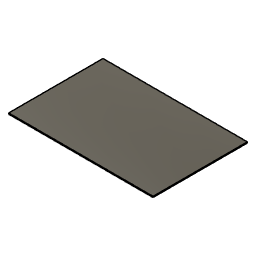
openbook_3D (Autodesk Fusion 360 archive; units mm, degrees)
design "screen"
Autodesk Fusion 360 part; units mm, degrees
box "BoxPrimitive1" add length 111.2 width 170.2 height 1.18 placed x (0, -1, 0) y (1, 0, 0) z (0, 0, 1) at (0.2, 0, 0)

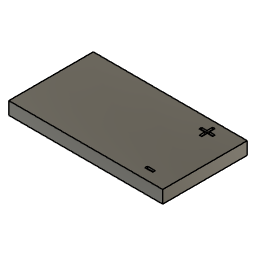
design "Battery"
part number: Configuration 1
Autodesk Fusion 360 part; units mm, degrees
box "BoxPrimitive1" add length 42 width 76.5 height 6.3 placed x (0, -1, 0) y (1, 0, 0) z (0, 0, 1) at (-66.5, 0, 0)
sketch "Sketch3" plane through (0, 0, 0) normal (0, 0, 1) x (1, 0, 0)
sketch "Sketch4" plane through (0, 0, 6.3) normal (0, 0, 1) x (-1, 0, 0)
  line L0 (66.5, 42) -> (-10, 42)
  line L1 (-10, 42) -> (-10, 0)
  line L2 (-10, 0) -> (66.5, 0)
  line L3 (66.5, 0) -> (66.5, 42)
  line L4 (0.5292, 2.4571) -> (7.6329, 2.6236) construction
  line L5 (7.6329, 2.6236) -> (7.4708, 9.5429) construction
  line L6 (7.4708, 9.5429) -> (0.3671, 9.3764) construction
  line L7 (0.3671, 9.3764) -> (0.5292, 2.4571) construction
  line L8 (1, 31) -> (8, 31) construction
  line L9 (8, 31) -> (8, 37) construction
  line L10 (8, 37) -> (1, 37) construction
  line L11 (1, 37) -> (1, 31) construction
  dimension "d8" = 10
  dimension "d9" = 10
  text T0 "+" font "Arial" height 10 align left top in box 7.1056 x 6.9211 at (0.5292, 2.4571) x (0.999726, 0.023427) y (-0.023427, 0.999726) spacing 1 kerned
extrude "Extrude1" cut sketch "Sketch4" against normal blind 1 text T0
sketch "Sketch5" plane through (0, 0, 6.3) normal (0, 0, 1) x (-1, 0, 0)
  line L0 (4.338, 5.6007) -> (4.4022, 2.8593)
  line L1 (4.4022, 2.8593) -> (3.2429, 2.8321)
  line L2 (3.2429, 2.8321) -> (3.1787, 5.5735)
  line L3 (3.1787, 5.5735) -> (0.4577, 5.5098)
  line L4 (0.4577, 5.5098) -> (0.4309, 6.6554)
  line L5 (0.4309, 6.6554) -> (3.1518, 6.7192)
  line L6 (3.1518, 6.7192) -> (3.088, 9.4401)
  line L7 (3.088, 9.4401) -> (4.2473, 9.4673)
  line L8 (4.2473, 9.4673) -> (4.3111, 6.7464)
  line L9 (4.3111, 6.7464) -> (7.0321, 6.8101)
  line L10 (7.0321, 6.8101) -> (7.0589, 5.6645)
  line L11 (7.0589, 5.6645) -> (4.338, 5.6007)
  line L12 (66.5, 42) -> (-10, 42)
  line L13 (-10, 42) -> (-10, 0)
  line L14 (-10, 0) -> (66.5, 0)
  line L15 (66.5, 0) -> (66.5, 42)
  line L16 (0, 30) -> (9, 30) construction
  line L17 (9, 30) -> (9, 37) construction
  line L18 (9, 37) -> (0, 37) construction
  line L19 (0, 37) -> (0, 30) construction
  dimension "d12" = 10
  text T0 "-" font "Arial" height 10 align left top in box 9 x 7 at (0, 30) x (1, 0) y (0, 1) spacing 1 kerned
extrude "Extrude2" cut sketch "Sketch5" against normal blind 1 text T0
